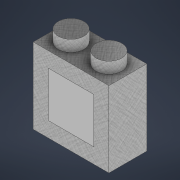
# Autodesk Inventor part: 110033226_ipt_22_塔樓牆壁
Saved by Autodesk Inventor 2022 (Build 260153000, 153)
## iProperties
Created: 2022-06-23
Part Number: 110033226_ipt_22_塔樓牆壁
Material: 一般
Document SubType Name: Modeling
Designer: User
Density: 1 g/cm^3
Appearance: 預設
Author: User
Autodesk Inventor part; units mm, degrees
ref_plane "YZ Plane" through (0, 0, 0) normal (1, 0, 0) x (0, 1, 0)
ref_plane "XZ Plane" through (0, 0, 0) normal (0, 1, 0) x (-1, 0, 0)
ref_plane "XY Plane" through (0, 0, 0) normal (0, 0, 1) x (1, 0, 0)
sketch "草圖2" plane through (0, 0, 0) normal (0, 1, 0) x (-1, 0, 0)
  line L0 (5, 2.5) -> (-5, 2.5)
  line L1 (-5, 2.5) -> (-5, -2.5)
  line L2 (-5, -2.5) -> (5, -2.5)
  line L3 (5, -2.5) -> (5, 2.5)
  circle A0 centre (2.5, 0) radius 1.7
  circle A1 centre (-2.5, 0) radius 1.7
  point P0 (0, 0)
  point P1 (5, 0)
  point P2 (0, -2.5)
  dimension "d0" = 10
  dimension "d1" = 5
  dimension "d2" = 3.4
  dimension "d3" = 2.5
  dimension "d4" = 2.5
  dimension "d7" = 5
  constraints: 8 end point, 2 centre point, 2 horizontal, 2 midpoint, 2 parallel, 1 horizontal alignment, 1 perpendicular, 1 vertical alignment, 2 other
  measures "d0" distance of L2.end L1.end
  measures "d1" distance of L1.end L0.end
  measures "d2" diameter of A0
  measures "d3" distance from line of L2 A0.centre
  measures "d4" distance from line of L3 A0.centre
  measures "d7" distance of A0.centre A1.centre
extrude "擠出1" add sketch "草圖2" along normal blind 10 contours L3 L2 L1 L0 | A0 | A1
extrude "擠出2" cut sketch "草圖2" along normal blind 1.5 contours A0 | A1
sketch "草圖3" plane through (0, 10, 0) normal (0, 1, 0) x (1, 0, 0)
  circle A0 centre (-2.5, 0) radius 1.7 projected
  circle A1 centre (2.5, 0) radius 1.7 projected
  point P0 (0, 0)
extrude "擠出3" add sketch "草圖3" along normal blind 1.5
sketch "草圖4" plane through (0, 0, 0) normal (0, 0, 1) x (1, 0, 0)
  line L0 (5, 10) -> (5, 0) projected
  line L1 (5, 0) -> (4.2, 0) projected
  line L2 (4.2, 0) -> (4.2, 1.5) projected
  line L3 (4.2, 1.5) -> (0.8, 1.5) projected
  line L4 (0.8, 1.5) -> (0.8, 0) projected
  line L5 (0.8, 0) -> (-0.8, 0) projected
  line L6 (-0.8, 0) -> (-0.8, 1.5) projected
  line L7 (-0.8, 1.5) -> (-4.2, 1.5) projected
  line L8 (-4.2, 1.5) -> (-4.2, 0) projected
  line L9 (-4.2, 0) -> (-5, 0) projected
  line L10 (-5, 0) -> (-5, 10) projected
  line L11 (-5, 10) -> (-4.2, 10) projected
  line L12 (-4.2, 10) -> (-4.2, 11.5) projected
  line L13 (-4.2, 11.5) -> (-0.8, 11.5) projected
  line L14 (-0.8, 11.5) -> (-0.8, 10) projected
  line L15 (-0.8, 10) -> (0.8, 10) projected
  line L16 (0.8, 10) -> (0.8, 11.5) projected
  line L17 (0.8, 11.5) -> (4.2, 11.5) projected
  line L18 (4.2, 11.5) -> (4.2, 10) projected
  line L19 (4.2, 10) -> (5, 10) projected
  line L20 (-3, 8) -> (3, 8)
  line L21 (3, 8) -> (3, 2)
  line L22 (3, 2) -> (-3, 2)
  line L23 (-3, 2) -> (-3, 8)
  line L24 (0, 10) -> (0, 0) construction
  line L25 (5, 0) -> (-5, 0) construction
  point P0 (0, 8)
  point P1 (3, 5)
  point P2 (5, 5)
  dimension "d18" = 6
  dimension "d19" = 6
  constraints: 10 end point, 4 midpoint, 2 parallel, 2 perpendicular, 1 horizontal, 1 horizontal alignment, 1 point on line
  measures "d18" distance of L21.end L22.end
  measures "d19" distance of L20.end L21.end
split_face "分割1"
